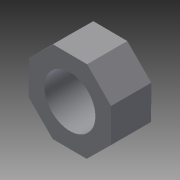
# Autodesk Inventor part: nut
Saved by Autodesk Inventor 2015 SP2 (Build 190223200, 223)
## iProperties
Created: 2016-09-06
Part Number: nut
Material: Generic
Document SubType Name: Modeling
Designer: jm799
Density: 1 g/cm^3
Appearance: Default
Author: jm799
Autodesk Inventor part; units mm, degrees
ref_plane "YZ Plane" through (0, 0, 0) normal (1, 0, 0) x (0, 1, 0)
ref_plane "XZ Plane" through (0, 0, 0) normal (0, 1, 0) x (-1, 0, 0)
ref_plane "XY Plane" through (0, 0, 0) normal (0, 0, 1) x (1, 0, 0)
sketch "Sketch1" plane through (0, 0, 0) normal (0, 1, 0) x (-1, 0, 0)
  circle A0 centre (0, 0) radius 0.95
  line L0 (0.6422, -1.5267) -> (-0.6254, -1.5337)
  line L1 (-0.6254, -1.5337) -> (-1.5267, -0.6422)
  line L2 (-1.5267, -0.6422) -> (-1.5337, 0.6254)
  line L3 (-1.5337, 0.6254) -> (-0.6422, 1.5267)
  line L4 (-0.6422, 1.5267) -> (0.6254, 1.5337)
  line L5 (0.6254, 1.5337) -> (1.5267, 0.6422)
  line L6 (1.5267, 0.6422) -> (1.5337, -0.6254)
  line L7 (1.5337, -0.6254) -> (0.6422, -1.5267)
  dimension "d0" = 1.9
  constraints: 16 end point, 2 coincident, 1 centre point, 17 other
  measures "d0" diameter of A0
extrude "Extrusion1" add sketch "Sketch1" along normal blind 1.5
body "Solid1"
